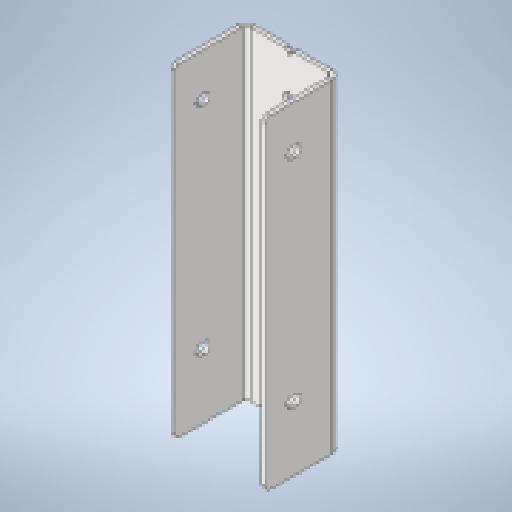
# Autodesk Inventor part: NDM 7.44 bracket middle
Saved by Autodesk Inventor 2025 (Build 290162010, 162A)
## iProperties
Created: 2023-07-04
Part Number: NDM 7.44 bracket middle
Material: Stainless Steel
Description: 2mm
Document SubType Name: Sheet Metal
Designer: DELL
Stock Number: NDM 7.1 папа ноги домкрат
Mass: 592.546 g
Surface Area: 766.755 cm^2
Volume: 74.0682 cm^3
Density: 8 g/cm^3
Flat Pattern Width: 10.7048 cm
Flat Pattern Length: 15 cm
Flat Pattern Area: 160.572 cm^2
Sheet Metal Rule: Default_mm
Sheet Metal Width: 107,048 mm
Sheet Metal Length: 150,000 mm
Sheet Metal Area: 16057,168 mm^2
Appearance: Default
Author: user
Revision Number: 8
Autodesk Inventor part; units mm, degrees
ref_plane "YZ Plane" through (0, 0, 0) normal (1, 0, 0) x (0, 1, 0)
ref_plane "XZ Plane" through (0, 0, 0) normal (0, 1, 0) x (-1, 0, 0)
ref_plane "XY Plane" through (0, 0, 0) normal (0, 0, 1) x (1, 0, 0)
sketch "Sketch1" plane through (0, 0, 0) normal (0, 0, 1) x (1, 0, 0)
  line L0 (-20, 75) -> (20, 75)
  line L1 (20, 75) -> (20, -75)
  line L2 (20, -75) -> (-20, -75)
  line L3 (-20, -75) -> (-20, 75)
  line L4 (-20, 75) -> (20, -75) construction
  line L5 (20, 75) -> (-20, -75) construction
  point P0 (0, 0)
  point P1 (0, 0)
  dimension "d0" = 40
  dimension "d1" = 150
  constraints: 12 end point, 2 midpoint, 1 coincident, 1 horizontal, 1 parallel, 1 perpendicular
  measures "d0" distance of L1.end L2.end
  measures "d1" distance of L2.end L0.start
extrude "Plate1" add sketch "Sketch1" along normal blind 2
sketch "Sketch2" plane through (-20, -75, 2) normal (-1, 0, 0) x (0, -1, 0)
  line L0 (-150, 0) -> (0, 0)
  line L1 (0, 0) -> (0, 33)
  line L2 (0, 33) -> (-150, 33)
  line L3 (-150, 33) -> (-150, 0)
  constraints: 6 end point, 1 horizontal, 1 perpendicular, 1 vertical
edge flange "Flange1" height 35 angle 90 thickness 2 bend radius 2 thickness toward (-1, 0, 0) relief tear relief width 2 relief depth 1 corner gap 2 corner form 0 edges at (-20, 0, 2) (20, 0, 2) wall of the first edge with corners at (-20, 75, 2) (-20, -75, 2) (-20, -75, 35) (-20, 75, 35)
bend "Bend1"
corner "Corner1"
sketch "Sketch3" plane through (0, 0, 0) normal (1, 0, 0) x (0, 1, 0)
  line L0 (-75, 4) -> (75, 4) projected
  line L1 (75, 35) -> (75, 4) projected
  line L2 (-75, 35) -> (75, 35) projected
  line L3 (-75, 4) -> (-75, 35) projected
  circle A0 centre (-55, 22) radius 2.5
  line L4 (-55, 22.75) -> (-55, 21.25) construction
  line L5 (-57.5, 22.75) -> (-57.5, 21.25)
  line L6 (-52.5, 21.25) -> (-52.5, 22.75)
  arc A1 (-52.5, 22.75) -> (-57.5, 22.75) centre (-55, 22.75) ccw
  arc A2 (-57.5, 21.25) -> (-52.5, 21.25) centre (-55, 21.25) ccw
  point P0 (0, 0)
  point P1 (-52.5, 22)
  point P2 (-57.5, 22)
  dimension "d13" = 5
  dimension "d14" = 13
  dimension "d15" = 20
  dimension "d29" = 1.5
  constraints: 8 end point, 5 tangent, 4 point on circle, 3 centre point, 1 coincident, 1 midpoint, 1 parallel, 1 vertical
  measures "d13" diameter of A0
  measures "d14" distance from line of A0.centre L2
  measures "d15" distance from line of L3 A0.centre
  measures "d29" distance of L4.start L4.end
extrude "Extrusion1" cut sketch "Sketch3" along normal through all both and the other way through all contours A0 | L6 A2 L5 A0 | A0 L5 A1 L6
pattern_linear "Rectangular Pattern2" count 2 spacing 100 along (0, 1, 0) of "Extrusion1"
fillet "Fillet1" radius 2 4 edges at (-21, -75, 35) (21, -75, 35) (-21, 75, 35) (21, 75, 35)
equation "\"d2\" = Thickness"
equation "\"d3\" = BendReliefWidth"
equation "\"d4\" = BendReliefDepth"
equation "\"d5\" = MinimumRemnant"
equation "\"d6\" = TransitionRadius"
equation "\"d9\" = BendRadius"
equation "\"d10\" = CornerReliefSize"
equation "\"d11\" = GapSize"
equation "\"d12\" = JacobiRadiusSize"
equation "\"BendRadius\" = Thickness"
equation "\"BendReliefWidth\" = Thickness"
equation "\"BendReliefDepth\" = 0.5 * Thickness"
equation "\"CornerReliefSize\" = 4 * Thickness"
equation "\"MinimumRemnant\" = 2 * Thickness"
equation "\"TransitionRadius\" = BendRadius"
equation "\"JacobiRadiusSize\" = BendRadius"
equation "\"GapSize\" = Thickness"
equation "\"Thickness\" = 2"
body "Solid1"
